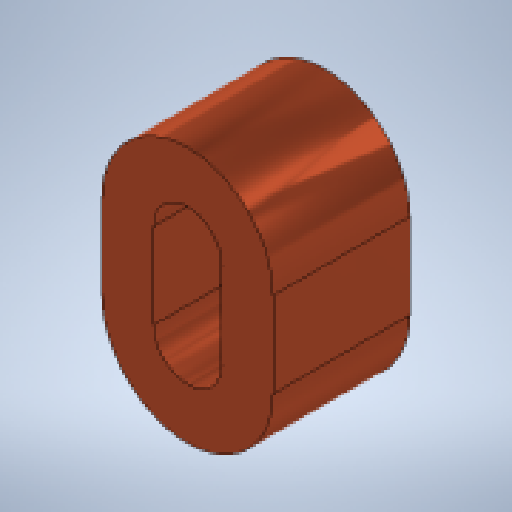
# Autodesk Inventor part: COILS
Saved by Autodesk Inventor 2023.2 (Build 272271000, 271)
## iProperties
Created: 2024-01-31
Part Number: COILS
Material: Copper
Document SubType Name: Modeling
Designer: Nathan Cai
Density: 8.94 g/cm^3
Appearance: Copper - Satin
Author: Nathan Cai
Autodesk Inventor part; units mm, degrees
ref_plane "YZ Plane" through (0, 0, 0) normal (1, 0, 0) x (0, 1, 0)
ref_plane "XZ Plane" through (0, 0, 0) normal (0, 1, 0) x (-1, 0, 0)
ref_plane "XY Plane" through (0, 0, 0) normal (0, 0, 1) x (1, 0, 0)
sketch "Sketch1" plane through (0, 0, 0) normal (0, 0, 1) x (1, 0, 0)
  line L0 (-1, -2.5) -> (1, -2.5)
  line L1 (1, -2.5) -> (1, 2.5)
  line L2 (1, 2.5) -> (-1, 2.5)
  line L3 (-1, 2.5) -> (-1, -2.5)
  line L4 (-1, -2.5) -> (1, 2.5) construction
  line L5 (1, -2.5) -> (-1, 2.5) construction
  line L6 (-2, -3.5) -> (2, -3.5)
  line L7 (2, -3.5) -> (2, 3.5)
  line L8 (2, 3.5) -> (-2, 3.5)
  line L9 (-2, 3.5) -> (-2, -3.5)
  line L10 (-2, -3.5) -> (2, 3.5) construction
  line L11 (2, -3.5) -> (-2, 3.5) construction
  point P0 (0, 0)
  point P1 (0, 0)
  dimension "d5" = 2
  dimension "d6" = 5
  dimension "d7" = 4
  dimension "d8" = 7
  constraints: 24 end point, 4 midpoint, 4 parallel, 2 horizontal, 2 perpendicular, 1 coincident, 1 other
  measures "d5" distance of L2.end L1.end
  measures "d6" distance of L1.end L0.end
  measures "d7" distance of L8.end L7.end
  measures "d8" distance of L7.end L6.end
extrude "Extrusion1" add sketch "Sketch1" along normal blind 4.5
fillet "Fillet1" radius 2 4 edges at (2, 3.5, 2.25) (-2, 3.5, 2.25) (2, -3.5, 2.25) (-2, -3.5, 2.25)
fillet "Fillet2" radius 0.5 4 edges at (-1, 2.5, 2.25) (1, 2.5, 2.25) (-1, -2.5, 2.25) (1, -2.5, 2.25)
body "Solid1"
